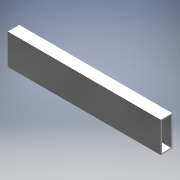
# Autodesk Inventor part: Extrusion Mid
Saved by Autodesk Inventor 2019.4 (Build 234330000, 330)
## iProperties
Created: 2020-01-07
Part Number: Extrusion Mid
Material: Aluminum 6061
Document SubType Name: Modeling
Designer: Mark
Mass: 673.15 g
Surface Area: 1676.65 cm^2
Volume: 249.315 cm^3
Density: 2.7 g/cm^3
Appearance: Aluminum - Flat
Author: Mark
Autodesk Inventor part; units mm, degrees
ref_plane "YZ Plane" through (0, 0, 0) normal (1, 0, 0) x (0, 1, 0)
ref_plane "XZ Plane" through (0, 0, 0) normal (0, 1, 0) x (-1, 0, 0)
ref_plane "XY Plane" through (0, 0, 0) normal (0, 0, 1) x (1, 0, 0)
sketch "Sketch1" plane through (0, 0, 0) normal (1, 0, 0) x (0, 1, 0)
  line L0 (-40, 15) -> (40, 15)
  line L1 (40, 15) -> (40, -15)
  line L2 (40, -15) -> (-40, -15)
  line L3 (-40, -15) -> (-40, 15)
  line L4 (-40, 15) -> (40, -15) construction
  line L5 (40, 15) -> (-40, -15) construction
  line L6 (-37, 12) -> (37, 12)
  line L7 (37, 12) -> (37, -12)
  line L8 (37, -12) -> (-37, -12)
  line L9 (-37, -12) -> (-37, 12)
  line L10 (-37, 12) -> (37, -12) construction
  line L11 (37, 12) -> (-37, -12) construction
  point P0 (0, 0)
  dimension "d0" = 80
  dimension "d1" = 30
  dimension "d2" = 74
  dimension "d3" = 24
  constraints: 24 end point, 4 midpoint, 4 parallel, 2 horizontal, 2 perpendicular
  measures "d0" distance of L1.end L2.end
  measures "d1" distance of L0.end L1.end
  measures "d2" distance of L7.end L8.end
  measures "d3" distance of L6.end L7.end
extrude "Extrusion1" add sketch "Sketch1" along normal blind 400
sketch "Sketch2" plane through (0, -40, -15) normal (0, -1, 0) x (1, 0, 0)
  circle A0 centre (40, 15) radius 2.75
  circle A1 centre (360, 15) radius 2.75
  line L0 (0, 30) -> (400, 30) projected
  line L1 (400, 30) -> (400, 0) projected
  line L2 (0, 0) -> (0, 30) projected
  point P0 (0, 15)
  dimension "d6" = 5.5
  dimension "d7" = 5.5
  dimension "d8" = 15
  dimension "d9" = 40
  dimension "d10" = 15
  dimension "d11" = 40
  constraints: 2 centre point
  measures "d6" diameter of A0
  measures "d7" diameter of A1
  measures "d8" distance from line of L0 A1.centre
  measures "d9" distance from line of L1 A1.centre
  measures "d10" distance from line of L0 A0.centre
  measures "d11" distance from line of L2 A0.centre
extrude "Extrusion2" cut sketch "Sketch2" against normal blind 80
body "Solid1"
